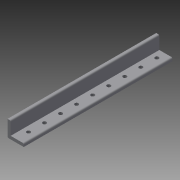
# Autodesk Inventor part: L Bracket with holes
Saved by Autodesk Inventor 2015 (Build 190159000, 159)
## iProperties
Created: 2014-11-21
Part Number: L Bracket with holes
Material: Generic
Document SubType Name: Modeling
Designer: willardw
Density: 1 g/cm^3
Appearance: Default
Author: willardw
Autodesk Inventor part; units mm, degrees
ref_plane "YZ Plane" through (0, 0, 0) normal (1, 0, 0) x (0, 1, 0)
ref_plane "XZ Plane" through (0, 0, 0) normal (0, 1, 0) x (-1, 0, 0)
ref_plane "XY Plane" through (0, 0, 0) normal (0, 0, 1) x (1, 0, 0)
sketch "Sketch1" plane through (0, 0, 0) normal (0, 0, 1) x (1, 0, 0)
  line L0 (52.418, 170.3116) -> (67.15, 170.3116)
  line L1 (67.15, 170.3116) -> (67.15, 167.2636)
  line L2 (51.148, 171.5816) -> (51.148, 186.3136)
  line L3 (51.148, 186.3136) -> (52.926, 186.3136)
  line L4 (54.196, 185.0436) -> (54.196, 173.3596)
  line L5 (67.15, 170.3116) -> (67.15, 172.0896)
  line L6 (65.88, 173.3596) -> (54.196, 173.3596)
  arc A0 (54.196, 185.0436) -> (52.926, 186.3136) centre (52.926, 185.0436) ccw
  arc A1 (67.15, 172.0896) -> (65.88, 173.3596) centre (65.88, 172.0896) ccw
  arc A2 (51.148, 171.5816) -> (52.418, 170.3116) centre (52.418, 171.5816) ccw
  point P0 (0, 0)
  point P1 (51.148, 170.3116)
  point P2 (54.196, 186.3136)
  point P3 (67.15, 173.3596)
  dimension "d0" = 16.002
  dimension "d1" = 3.048
  dimension "d2" = 16.002
  dimension "d3" = 3.048
  dimension "d4" = 3.048
  dimension "d5" = 1.27
  dimension "d6" = 1.27
  constraints: 14 end point, 6 point on circle, 6 point on line, 6 tangent, 3 centre point, 3 perpendicular, 2 vertical, 1 equal radius, 1 horizontal, 1 parallel
  measures "d0" distance of point (51.148, 170.312) L0.end
  measures "d1" distance of L0.end L1.end
  measures "d2" distance of point (51.148, 170.312) L2.end
  measures "d3" distance of L2.end point (54.196, 186.314)
  measures "d4" distance of L0.end point (67.15, 173.36)
  measures "d5" radius of A0
  measures "d6" radius of A1
extrude "Extrusion1" add sketch "Sketch1" along normal blind 146.304
sketch "Sketch3" plane through (54.196, 173.3596, 0) normal (0, 1, 0) x (1, 0, 0)
  line L0 (0.9375, 6.2475) -> (13.2819, 6.2475)
  line L1 (12.954, 0) -> (-1.778, 0) projected
  line L2 (5.588, 0) -> (5.588, -6.1341)
  line L3 (-1.778, -146.304) -> (12.954, -146.304) projected
  circle A0 centre (5.588, -7.9756) radius 1.8415
  line L4 (5.588, -7.9756) -> (5.588, -130.5306)
  circle A1 centre (5.588, -134.2136) radius 1.8415
  point P0 (-54.196, 0)
  dimension "d31" = 12.3444
  dimension "d32" = 6.1341
  dimension "d38" = 122.555
  constraints: 6 end point, 2 vertical, 1 centre point, 1 coincident, 1 horizontal, 1 midpoint, 1 vertical alignment, 2 other
  measures "d31" distance of L0.start L0.end
  measures "d32" distance of L2.start L2.end
  measures "d38" distance of L4.start L4.end
extrude "Extrusion6" cut sketch "Sketch3" against normal blind 69.85
sketch "Sketch4" plane through (54.196, 173.3596, 0) normal (0, 1, 0) x (1, 0, 0)
  circle A0 centre (5.588, -7.9756) radius 1.8415 projected
  line L0 (5.588, -25.6184) -> (6.1855, -25.6184)
  circle A1 centre (5.588, -23.7769) radius 1.8415
  circle A2 centre (5.588, -39.5757) radius 1.8415
  circle A3 centre (5.588, -55.3745) radius 1.8415
  circle A4 centre (5.588, -71.1733) radius 1.8415
  circle A5 centre (5.588, -86.9721) radius 1.8415
  circle A6 centre (5.588, -102.7709) radius 1.8415
  circle A7 centre (5.588, -118.5697) radius 1.8415
  point P0 (-54.196, 0)
  constraints: 6 centre point, 2 end point, 1 horizontal, 1 vertical alignment, 2 other
extrude "Extrusion7" cut sketch "Sketch4" against normal blind 34.925 contours A1 | A2 | A3 | A4 | A5 | A6 | A7
body "Solid1"
